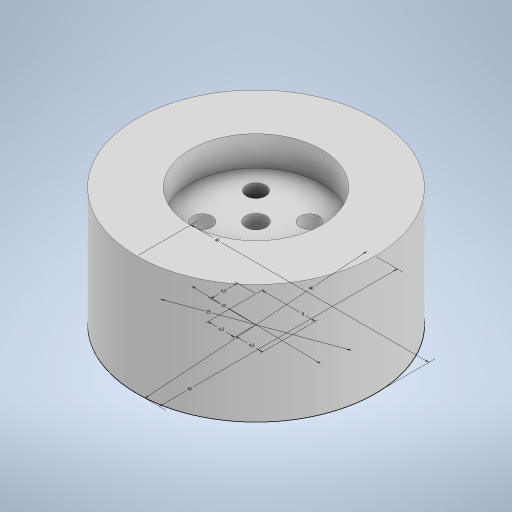
# Autodesk Inventor part: wheel
Saved by Autodesk Inventor 2023 (Build 270158000, 158)
## iProperties
Created: 2023-03-02
Part Number: wheel
Material: Generic
Document SubType Name: Modeling
Designer: KMRro
Density: 1 g/cm^3
Appearance: Default
Author: KMRro
Autodesk Inventor part; units mm, degrees
ref_plane "YZ Plane" through (0, 0, 0) normal (1, 0, 0) x (0, 1, 0)
ref_plane "XZ Plane" through (0, 0, 0) normal (0, 1, 0) x (-1, 0, 0)
ref_plane "XY Plane" through (0, 0, 0) normal (0, 0, 1) x (1, 0, 0)
sketch "Szkic1" plane through (0, 0, 0) normal (0, 1, 0) x (-1, 0, 0)
  circle A0 centre (0, 0) radius 20
  circle A1 centre (0, 0) radius 12.5
  circle A2 centre (0, 0) radius 11
  line L0 (20, 0) -> (-20, 0)
  line L1 (0, 20) -> (0, -20)
  point P0 (4.5, -4.5)
  point P1 (-4.5, -4.5)
  point P2 (4.5, 4.5)
  point P3 (-4.5, 4.5)
  dimension "d0" = 40
  dimension "d1" = 25
  dimension "d2" = 22
  dimension "d3" = 40
  dimension "d6" = 40
  dimension "d35" = 9
  dimension "d36" = 4.5
  dimension "d37" = 4.5
  dimension "d38" = 4.5
  constraints: 4 coincident, 4 end point, 4 point on circle, 3 centre point, 2 midpoint, 2 symmetric about line, 1 horizontal, 1 vertical
  measures "d0" diameter of A0
  measures "d1" diameter of A1
  measures "d2" diameter of A2
  measures "d3" distance of L0.start L0.end
  measures "d6" distance of L1.start L1.end
  measures "d35" distance of point (-4.5, -4.5) point (4.5, -4.5)
  measures "d36" horizontal distance of point (0, 0) point (4.5, -4.5)
  measures "d37" horizontal distance of point (0, 0) point (-4.5, -4.5)
  measures "d38" horizontal distance of point (0, 0) point (4.5, -4.5)
extrude "Wyciągnięcie proste1" add sketch "Szkic1" along normal blind 20 contours L0 A1 L1 A0 | A0 L1 A1 L0 | L1 A1 L0 A0 | A0 L0 A1 L1 | L0 A2 L1 A1 | A1 L1 A2 L0 | L1 A2 L0 A1 | A1 L0 A2 L1
extrude "Wyciągnięcie proste2" add sketch "Szkic1" along normal blind 15 contours L0 L1 A2 | A2 L1 L0 | L1 L0 A2 | A2 L0 L1
hole "Otwór2" at (0, 0, 0) direction (0, 1, 0) diameter 3.4 end through all clearance for "Countersunk Flat Head Screw ISO 2009/7046" size "M3" standard "ISO"
hole "Hole4" at (-4.5, 0, -4.5) at (4.5, 0, -4.5) at (-4.5, 0, 4.5) at (4.5, 0, 4.5) direction (0, 1, 0) diameter 3.2 depth 30 clearance for "Slotted Cheese Head Screw ISO 1207" size "M3" standard "ISO"
